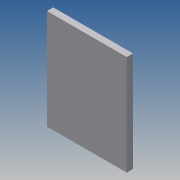
# Autodesk Inventor part: Tastatur
Saved by Autodesk Inventor 2019 (Build 230136000, 136)
## iProperties
Created: 2022-10-28
Part Number: Tastatur
Material: Generisch
Document SubType Name: Modeling
Designer: Dominik Schmidt
Density: 1 g/cm^3
Appearance: Weiß
Author: Dominik Schmidt
Autodesk Inventor part; units mm, degrees
ref_plane "YZ Plane" through (0, 0, 0) normal (1, 0, 0) x (0, 1, 0)
ref_plane "XZ Plane" through (0, 0, 0) normal (0, 1, 0) x (-1, 0, 0)
ref_plane "XY Plane" through (0, 0, 0) normal (0, 0, 1) x (1, 0, 0)
sketch "Skizze1" plane through (0, 0, 0) normal (0, 0, 1) x (1, 0, 0)
  line L0 (-25.5, 32) -> (25.5, 32)
  line L1 (25.5, 32) -> (25.5, -32)
  line L2 (25.5, -32) -> (-25.5, -32)
  line L3 (-25.5, -32) -> (-25.5, 32)
  line L4 (-25.5, 32) -> (25.5, -32) construction
  line L5 (25.5, 32) -> (-25.5, -32) construction
  point P0 (0, 0)
  dimension "d0" = 51
  dimension "d1" = 64
  constraints: 12 end point, 2 midpoint, 2 parallel, 1 horizontal, 1 perpendicular
  measures "d0" distance of L1.end L2.end
  measures "d1" distance of L0.end L1.end
extrude "Extrusion1" add sketch "Skizze1" along normal blind 4
